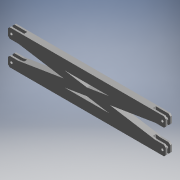
# Autodesk Inventor part: stabilizer
Saved by Autodesk Inventor 2019 (Build 230136000, 136)
## iProperties
Part Number: stabilizer
Material: Generic
Document SubType Name: Modeling
Designer: Jorge
Appearance: Default
Author: Jorge
## iProperties of the stored document stabilizer_3DPrint.ipt
Part Number: stabilizer_3DPrint
Material: Generic
Document SubType Name: Modeling
Designer: Jorge
Appearance: Default
Author: Jorge
Autodesk Inventor part; units mm, degrees
ref_plane "YZ Plane" through (0, 0, 0) normal (1, 0, 0) x (0, 1, 0)
ref_plane "XZ Plane" through (0, 0, 0) normal (0, 1, 0) x (-1, 0, 0)
ref_plane "XY Plane" through (0, 0, 0) normal (0, 0, 1) x (1, 0, 0)
sketch "Sketch1" plane through (0, 0, 0) normal (0, 0, 1) x (1, 0, 0)
  circle A0 centre (-91.5, 0) radius 1.5
  circle A1 centre (91.5, 0) radius 1.5
  line L0 (0, -71.4835) -> (0, 99.0835) construction
  line L1 (95.5, 4) -> (95.5, -4)
  line L2 (93.5, -6) -> (-93.5, -6)
  line L3 (-95.5, -4) -> (-95.5, 4)
  line L4 (-207.6267, 0) -> (207.6267, 0) construction
  line L5 (-93.5, 6) -> (-95.5, 4)
  line L6 (-93.5, -6) -> (-95.5, -4)
  line L7 (95.5, -4) -> (93.5, -6)
  line L8 (93.5, 6) -> (95.5, 4)
  line L9 (-148.3048, 15) -> (148.3048, 15) construction
  circle A2 centre (-91.5, 30) radius 1.5
  circle A3 centre (91.5, 30) radius 1.5
  line L10 (0, 101.4835) -> (0, -69.0835)
  line L11 (95.5, 26) -> (95.5, 34)
  line L12 (93.5, 36) -> (-93.5, 36)
  line L13 (-95.5, 34) -> (-95.5, 26)
  line L14 (-93.5, 24) -> (-95.5, 26)
  line L15 (-93.5, 36) -> (-95.5, 34)
  line L16 (95.5, 34) -> (93.5, 36)
  line L17 (93.5, 24) -> (95.5, 26)
  line L18 (87.5822, -3.9178) -> (95.4178, 3.9178) construction
  line L19 (-83, 6) -> (-27.9101, 15)
  line L20 (0, 19.5597) -> (27.1798, 24)
  line L21 (83, 24) -> (27.9101, 15)
  line L22 (0, 10.4403) -> (-27.1798, 6)
  line L23 (83, 6) -> (27.9101, 15)
  line L24 (0, 19.5597) -> (-27.1798, 24)
  line L25 (-83, 24) -> (-27.9101, 15)
  line L26 (0, 10.4403) -> (27.1798, 6)
  line L27 (-93.5, 24) -> (-83, 24)
  line L28 (-93.5, 6) -> (-83, 6)
  line L29 (-27.1798, 6) -> (27.1798, 6)
  line L30 (83, 6) -> (93.5, 6)
  line L31 (-27.1798, 24) -> (27.1798, 24)
  line L32 (83, 24) -> (93.5, 24)
  point P0 (0, 0)
  point P1 (-95.5, 6)
  point P2 (95.5, -6)
  point P3 (95.5, 6)
  point P4 (-95.5, -6)
  point P5 (0, 30)
  point P6 (-95.5, 24)
  point P7 (95.5, 36)
  point P8 (95.5, 24)
  point P9 (-95.5, 36)
  dimension "d0" = 3
  dimension "d1" = 3
  dimension "d2" = 183
  dimension "d4" = 4
  dimension "d10" = 2
  dimension "d11" = 2
  dimension "d12" = 2
  dimension "d13" = 2
  dimension "d14" = 2
  dimension "d15" = 2
  dimension "d16" = 2
  dimension "d17" = 2
  dimension "d18" = 30
  dimension "d20" = 12
  dimension "d21" = 12
  dimension "d22" = 12
  dimension "d23" = 10.5
  dimension "d24" = 10.5
  dimension "d25" = 9
  dimension "d26" = 9
  dimension "d27" = 9
  dimension "d28" = 9
  dimension "d29" = 12
  constraints: 62 end point, 20 symmetric about line, 15 point on line, 7 parallel, 4 centre point, 4 collinear, 4 horizontal, 3 perpendicular, 2 coincident, 1 midpoint, 4 other
  measures "d0" diameter of A0
  measures "d1" diameter of A1
  measures "d2" distance of A1.centre A0.centre
  measures "d4" distance from line of A0.centre L3
  measures "d10" distance of L5.start point (-95.5, 6)
  measures "d11" distance of L3.end point (-95.5, 6)
  measures "d12" distance of L2.end point (-95.5, -6)
  measures "d13" distance of L3.start point (-95.5, -6)
  measures "d14" distance of L1.end point (95.5, -6)
  measures "d15" distance of L2.start point (95.5, -6)
  measures "d16" distance of L8.start point (95.5, 6)
  measures "d17" distance of L1.start point (95.5, 6)
  measures "d18" distance of A0.centre A2.centre
  measures "d20" distance between parallel lines of L2 L30
  measures "d21" distance between parallel lines of L2 L29
  measures "d22" distance between parallel lines of L2 L28
  measures "d23" distance of L14.start L25.start
  measures "d24" distance of L21.start L17.start
  measures "d25" distance between parallel lines of L24 L25
  measures "d26" distance between parallel lines of L22 L19
  measures "d27" distance between parallel lines of L23 L26
  measures "d28" distance between parallel lines of L21 L20
  measures "d29" distance between parallel lines of L12 L31
extrude "Extrusion2" add sketch "Sketch1" along normal blind 7.6 contours L1 L7 L2 L10 L29 L26 L20 L31 L12 L16 L11 L17 L32 L21 L23 L30 L8 | L2 L6 L3 L5 L28 L19 L25 L27 L14 L13 L15 L12 L10 L31 L24 L22 L29
sketch "Sketch2" plane through (-93.5, 36, 0) normal (0, 1, 0) x (1, 0, 0)
  line L0 (187, 0) -> (0, 0) construction
  line L1 (0, 0) -> (0, -7.6) construction
  line L2 (187, -7.6) -> (0, -7.6) construction
  line L3 (187, 0) -> (187, -7.6) construction
  line L4 (0, 0) -> (0, -7.6) construction
  line L5 (0, -3.8) -> (187, -3.8) construction
  line L6 (-2, -2) -> (15.5, -2)
  line L7 (15.5, -2) -> (15.5, -5.6)
  line L8 (15.5, -5.6) -> (-2, -5.6)
  line L9 (-2, -5.6) -> (-2, -2)
  line L10 (-2, 0) -> (-2, -7.6) construction
  line L11 (93.5, 0) -> (93.5, -7.6) construction
  line L12 (0, -7.6) -> (187, -7.6) construction
  line L13 (187, 0) -> (187, -7.6) construction
  line L14 (187, 0) -> (187, -7.6) construction
  line L15 (187, -3.8) -> (0, -3.8) construction
  line L16 (189, -2) -> (171.5, -2)
  line L17 (171.5, -2) -> (171.5, -5.6)
  line L18 (171.5, -5.6) -> (189, -5.6)
  line L19 (189, -5.6) -> (189, -2)
  line L20 (189, 0) -> (189, -7.6) construction
  dimension "d32" = 3.6
  dimension "d33" = 17.5
  constraints: 28 end point, 8 symmetric about line, 3 midpoint, 2 parallel, 1 collinear, 1 horizontal, 1 perpendicular, 1 other
  measures "d32" distance between parallel lines of L8 L6
  measures "d33" distance between parallel lines of L9 L7
extrude "Extrusion3" cut sketch "Sketch2" against normal through all
equation "\"d11\" = d10"
equation "\"d13\" = d12"
equation "\"d14\" = d12"
equation "\"d15\" = d14"
equation "\"d16\" = d12"
equation "\"d17\" = d16"
body "Solid2"
